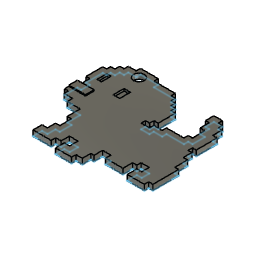
pixel_art_dog_keychain (Autodesk Fusion 360 design; units mm, degrees)
Autodesk Fusion 360 part; units mm, degrees
sketch "Dog_body" plane through (0, 0, 0) normal (0, 0, 1) x (1, 0, 0)
  line L0 (-5.9546, 3.7769) -> (-5.6, 3.7769)
  line L1 (-5.6, 3.7769) -> (-5.6, 4.1551)
  line L2 (-5.6, 4.1551) -> (-5.2, 4.1551)
  line L3 (-5.2, 4.1551) -> (-5.2, 4.6)
  line L4 (-5.2, 4.6) -> (-4.8, 4.6)
  line L5 (-4.8, 4.6) -> (-4.8, 5)
  line L6 (-4.8, 5) -> (-4.0585, 5)
  line L7 (-4.0585, 5) -> (-4.0585, 5.4)
  line L8 (-4.0585, 5.4) -> (-2.4, 5.4)
  line L9 (-2.4, 5.4) -> (-2.4, 5)
  line L10 (-2.4, 5) -> (-0.4, 5)
  line L11 (-0.4, 5) -> (-0.4, 4.6)
  line L12 (-5.9546, 3.7769) -> (-5.9546, 2.2)
  line L13 (-5.9546, 2.2) -> (-5.6, 2.2)
  line L14 (-5.6, 2.2) -> (-5.6, 1.4)
  line L15 (-5.6, 1.4) -> (-5.9546, 1.4)
  line L16 (-5.9546, 1.4) -> (-5.9546, 0.2)
  line L17 (-5.9546, 0.2) -> (-5.6, 0.2)
  line L18 (-5.6, 0.2) -> (-5.6, -0.2)
  line L19 (-5.6, -0.2) -> (-4.8, -0.2)
  line L20 (-4.8, -0.2) -> (-4.8, -0.7)
  line L21 (-4.8, -0.7) -> (-3.6, -0.7)
  line L22 (-3.6, -0.7) -> (-3.6, -1.9)
  line L23 (-3.6, -1.9) -> (-3.2, -1.9)
  line L24 (-3.2, -1.9) -> (-3.2, -3)
  line L25 (-3.2, -3) -> (-3.6, -3)
  line L26 (-3.6, -3) -> (-3.6, -3.7529)
  line L27 (-3.6, -3.7529) -> (-4.1, -3.7529)
  line L28 (-4.1, -3.7529) -> (-4.1, -4.6)
  line L29 (-4.1, -4.6) -> (-2.4, -4.6)
  line L30 (-2.4, -4.6) -> (-2.4, -4.1765)
  line L31 (-2.4, -4.1765) -> (-1.9, -4.1765)
  line L32 (-1.9, -4.1765) -> (-1.9, -3.4)
  line L33 (-1.9, -3.4) -> (-1.1, -3.4)
  line L34 (-1.1, -3.4) -> (-1.1, -4.1765)
  line L35 (-1.1, -4.1765) -> (-1.6, -4.1765)
  line L36 (-1.6, -4.1765) -> (-1.6, -5)
  line L37 (-1.6, -5) -> (-0.1, -5)
  line L38 (-0.1, -5) -> (-0.1, -4.5882)
  line L39 (-0.1, -4.5882) -> (0.5, -4.5882)
  line L40 (0.5, -4.5882) -> (0.5, -3.8)
  line L41 (5.1495, 3.3539) -> (5.1495, 1.4)
  line L42 (5.1495, 1.4) -> (4.8, 1.4)
  line L43 (4.8, 1.4) -> (4.8, 1)
  line L44 (4.8, 1) -> (5.1495, 1)
  line L45 (5.1495, 1) -> (5.1495, 0.2)
  line L46 (5.1495, 0.2) -> (5.5479, 0.2)
  line L47 (5.5479, 0.2) -> (5.5479, -1)
  line L48 (5.5479, -1) -> (5.9, -1)
  line L49 (5.9, -1) -> (5.9, -3.4)
  line L50 (-0.4, 4.6) -> (0, 4.6)
  line L51 (0, 4.6) -> (0, 4.2)
  line L52 (0, 4.2) -> (0.4, 4.2)
  line L53 (0.4, 4.2) -> (0.4, 3.8)
  line L54 (0.4, 3.8) -> (0.8, 3.8)
  line L55 (0.8, 3.8) -> (0.8, 3.4)
  line L56 (0.8, 3.4) -> (1.2, 3.4)
  line L57 (1.2, 3.4) -> (1.2, 1.8)
  line L58 (1.2, 1.8) -> (0.8, 1.8)
  line L59 (0.8, 1.8) -> (0.8, 1.4)
  line L60 (0.8, 1.4) -> (0.4, 1.4)
  line L61 (0.4, 1.4) -> (0.4, 1)
  line L62 (0.4, 1) -> (1.1786, 1)
  line L63 (1.1786, 1) -> (1.1786, 1.4)
  line L64 (1.1786, 1.4) -> (1.9689, 1.4)
  line L65 (1.9689, 1.4) -> (1.9689, 1.8)
  line L66 (1.9689, 1.8) -> (3.6, 1.8)
  line L67 (3.6, 1.8) -> (3.6, 2.2)
  line L68 (3.6, 2.2) -> (4, 2.2)
  line L69 (4, 2.2) -> (4, 3.3596)
  line L70 (4, 3.3596) -> (3.5503, 3.3596)
  line L71 (3.5503, 3.3596) -> (3.5503, 4.2)
  line L72 (3.5503, 4.2) -> (3.2, 4.2)
  line L73 (3.2, 4.2) -> (3.2, 5)
  line L74 (3.2, 5) -> (4, 5)
  line L75 (4, 5) -> (4, 4.6)
  line L76 (4, 4.6) -> (4.4, 4.6)
  line L77 (4.4, 4.6) -> (4.4, 4.2)
  line L78 (4.4, 4.2) -> (4.7373, 4.2)
  line L79 (4.7373, 4.2) -> (4.7373, 3.4)
  line L80 (4.7373, 3.4) -> (4.7373, 3.3539)
  line L81 (4.7373, 3.3539) -> (5.1495, 3.3539)
  line L82 (0.5, -3.8) -> (0.8, -3.8)
  line L83 (0.8, -3.8) -> (0.8, -3)
  line L84 (0.8, -3) -> (1.5654, -3)
  line L85 (1.5654, -3) -> (1.5654, -3.5)
  line L86 (1.5654, -3.5) -> (3.2, -3.5)
  line L87 (3.2, -3.5) -> (3.2, -2.6)
  line L88 (3.2, -2.6) -> (3.6, -2.6)
  line L89 (3.6, -2.6) -> (3.6, -2.2)
  line L90 (3.6, -2.2) -> (4.3564, -2.2)
  line L91 (4.3564, -2.2) -> (4.3564, -2.9)
  line L92 (4.3564, -2.9) -> (3.9, -2.9)
  line L93 (3.9, -2.9) -> (3.9, -3.8)
  line L94 (3.9, -3.8) -> (5.5, -3.8)
  line L95 (5.5, -3.4) -> (5.9, -3.4)
  line L96 (5.5, -3.4) -> (5.5, -3.8)
  constraint horizontal L0
  constraint perpendicular L0 L1
  constraint perpendicular L1 L2
  constraint perpendicular L2 L3
  constraint perpendicular L3 L4
  constraint perpendicular L4 L5
  constraint perpendicular L3 L6
  constraint perpendicular L6 L7
  constraint perpendicular L7 L8
  constraint perpendicular L8 L9
  constraint perpendicular L9 L10
  constraint perpendicular L10 L11
  constraint perpendicular L0 L12
  constraint perpendicular L12 L13
  constraint perpendicular L0 L14
  constraint perpendicular L14 L15
  constraint perpendicular L0 L16
  constraint perpendicular L14 L17
  constraint perpendicular L0 L18
  constraint perpendicular L18 L19
  constraint perpendicular L19 L20
  constraint perpendicular L20 L21
  constraint perpendicular L21 L22
  constraint perpendicular L22 L23
  constraint perpendicular L23 L24
  constraint perpendicular L24 L25
  constraint perpendicular L25 L26
  constraint perpendicular L24 L27
  constraint perpendicular L27 L28
  constraint perpendicular L28 L29
  constraint perpendicular L29 L30
  constraint perpendicular L30 L31
  constraint perpendicular L31 L32
  constraint perpendicular L32 L33
  constraint perpendicular L31 L34
  constraint perpendicular L34 L35
  constraint perpendicular L35 L36
  constraint perpendicular L36 L37
  constraint perpendicular L37 L38
  constraint perpendicular L38 L39
  constraint perpendicular L39 L40
  constraint vertical L41
  constraint perpendicular L41 L42
  constraint perpendicular L42 L43
  constraint perpendicular L43 L44
  constraint perpendicular L44 L45
  constraint perpendicular L45 L46
  constraint perpendicular L46 L47
  constraint perpendicular L47 L48
  constraint perpendicular L46 L49
  constraint perpendicular L11 L50
  constraint perpendicular L50 L51
  constraint perpendicular L51 L52
  constraint perpendicular L52 L53
  constraint perpendicular L53 L54
  constraint perpendicular L52 L55
  constraint perpendicular L55 L56
  constraint perpendicular L56 L57
  constraint perpendicular L57 L58
  constraint perpendicular L58 L59
  constraint perpendicular L59 L60
  constraint perpendicular L60 L61
  constraint perpendicular L59 L62
  constraint perpendicular L62 L63
  constraint perpendicular L63 L64
  constraint perpendicular L62 L65
  constraint perpendicular L65 L66
  constraint perpendicular L66 L67
  constraint perpendicular L67 L68
  constraint perpendicular L68 L69
  constraint perpendicular L67 L70
  constraint perpendicular L70 L71
  constraint perpendicular L71 L72
  constraint perpendicular L72 L73
  constraint perpendicular L73 L74
  constraint perpendicular L72 L75
  constraint perpendicular L75 L76
  constraint perpendicular L76 L77
  constraint perpendicular L77 L78
  constraint perpendicular L76 L79
  constraint perpendicular L76 L80
  constraint perpendicular L41 L81
  constraint perpendicular L40 L82
  constraint perpendicular L82 L83
  constraint perpendicular L83 L84
  constraint perpendicular L84 L85
  constraint perpendicular L85 L86
  constraint perpendicular L86 L87
  constraint perpendicular L87 L88
  constraint perpendicular L86 L89
  constraint perpendicular L89 L90
  constraint perpendicular L86 L91
  constraint perpendicular L91 L92
  constraint perpendicular L92 L93
  constraint perpendicular L91 L94
  constraint perpendicular L49 L95
  constraint perpendicular L94 L96
extrude "Extrude1" add sketch "Dog_body" along normal blind 0.5
sketch "Dog_eyes" plane through (0, 0, 0.5) normal (0, 0, 1) x (-1, 0, 0)
  line L0 (5.9546, -3.7769) -> (5.9546, -2.2)
  line L1 (5.9546, -2.2) -> (5.6, -2.2)
  line L2 (5.6, -2.2) -> (5.6, -1.4)
  line L3 (5.6, -1.4) -> (5.9546, -1.4)
  line L4 (5.9546, -1.4) -> (5.9546, -0.2)
  line L5 (5.9546, -0.2) -> (5.6, -0.2)
  line L6 (5.6, -0.2) -> (5.6, 0.2)
  line L7 (5.6, 0.2) -> (4.8, 0.2)
  line L8 (4.8, 0.2) -> (4.8, 0.7)
  line L9 (4.8, 0.7) -> (3.6, 0.7)
  line L10 (3.6, 0.7) -> (3.6, 1.9)
  line L11 (3.6, 1.9) -> (3.2, 1.9)
  line L12 (3.2, 1.9) -> (3.2, 3)
  line L13 (3.2, 3) -> (3.6, 3)
  line L14 (3.6, 3) -> (3.6, 3.7529)
  line L15 (3.6, 3.7529) -> (4.1, 3.7529)
  line L16 (4.1, 3.7529) -> (4.1, 4.6)
  line L17 (4.1, 4.6) -> (2.4, 4.6)
  line L18 (2.4, 4.6) -> (2.4, 4.1765)
  line L19 (2.4, 4.1765) -> (1.9, 4.1765)
  line L20 (1.9, 4.1765) -> (1.9, 3.4)
  line L21 (1.9, 3.4) -> (1.1, 3.4)
  line L22 (1.1, 3.4) -> (1.1, 4.1765)
  line L23 (1.1, 4.1765) -> (1.6, 4.1765)
  line L24 (1.6, 4.1765) -> (1.6, 5)
  line L25 (1.6, 5) -> (0.1, 5)
  line L26 (0.1, 5) -> (0.1, 4.5882)
  line L27 (0.1, 4.5882) -> (-0.5, 4.5882)
  line L28 (-0.5, 4.5882) -> (-0.5, 3.8)
  line L29 (-0.5, 3.8) -> (-0.8, 3.8)
  line L30 (-0.8, 3.8) -> (-0.8, 3)
  line L31 (-0.8, 3) -> (-1.5654, 3)
  line L32 (-1.5654, 3) -> (-1.5654, 3.5)
  line L33 (-1.5654, 3.5) -> (-3.2, 3.5)
  line L34 (-3.2, 3.5) -> (-3.2, 2.6)
  line L35 (-3.2, 2.6) -> (-3.6, 2.6)
  line L36 (-3.6, 2.6) -> (-3.6, 2.2)
  line L37 (-3.6, 2.2) -> (-4.3564, 2.2)
  line L38 (-4.3564, 2.2) -> (-4.3564, 2.9)
  line L39 (-4.3564, 2.9) -> (-3.9, 2.9)
  line L40 (-3.9, 2.9) -> (-3.9, 3.8)
  line L41 (-3.9, 3.8) -> (-5.5, 3.8)
  line L42 (-5.5, 3.8) -> (-5.5, 3.4)
  line L43 (-5.5, 3.4) -> (-5.9, 3.4)
  line L44 (-5.9, 3.4) -> (-5.9, 1)
  line L45 (-5.9, 1) -> (-5.5479, 1)
  line L46 (-5.5479, 1) -> (-5.5479, -0.2)
  line L47 (-5.5479, -0.2) -> (-5.1495, -0.2)
  line L48 (-5.1495, -0.2) -> (-5.1495, -1)
  line L49 (-5.1495, -1) -> (-4.8, -1)
  line L50 (-4.8, -1) -> (-4.8, -1.4)
  line L51 (-4.8, -1.4) -> (-5.1495, -1.4)
  line L52 (-5.1495, -1.4) -> (-5.1495, -3.3539)
  line L53 (-5.1495, -3.3539) -> (-4.7373, -3.3539)
  line L54 (-4.7373, -3.3539) -> (-4.7373, -4.2)
  line L55 (-4.7373, -4.2) -> (-4.4, -4.2)
  line L56 (-4.4, -4.2) -> (-4.4, -4.6)
  line L57 (-4.4, -4.6) -> (-4, -4.6)
  line L58 (-4, -4.6) -> (-4, -5)
  line L59 (-4, -5) -> (-3.2, -5)
  line L60 (-3.2, -5) -> (-3.2, -4.2)
  line L61 (-3.2, -4.2) -> (-3.5503, -4.2)
  line L62 (-3.5503, -4.2) -> (-3.5503, -3.3596)
  line L63 (-3.5503, -3.3596) -> (-4, -3.3596)
  line L64 (-4, -3.3596) -> (-4, -2.2)
  line L65 (-4, -2.2) -> (-3.6, -2.2)
  line L66 (-3.6, -2.2) -> (-3.6, -1.8)
  line L67 (-3.6, -1.8) -> (-1.9689, -1.8)
  line L68 (-1.9689, -1.8) -> (-1.9689, -1.4)
  line L69 (-1.9689, -1.4) -> (-1.1786, -1.4)
  line L70 (-1.1786, -1.4) -> (-1.1786, -1)
  line L71 (-1.1786, -1) -> (-0.4, -1)
  line L72 (-0.4, -1) -> (-0.4, -1.4)
  line L73 (-0.4, -1.4) -> (-0.8, -1.4)
  line L74 (-0.8, -1.4) -> (-0.8, -1.8)
  line L75 (-0.8, -1.8) -> (-1.2, -1.8)
  line L76 (-1.2, -1.8) -> (-1.2, -3.4)
  line L77 (-1.2, -3.4) -> (-0.8, -3.4)
  line L78 (-0.8, -3.4) -> (-0.8, -3.8)
  line L79 (-0.8, -3.8) -> (-0.4, -3.8)
  line L80 (-0.4, -3.8) -> (-0.4, -4.2)
  line L81 (-0.4, -4.2) -> (0, -4.2)
  line L82 (0, -4.2) -> (0, -4.6)
  line L83 (0, -4.6) -> (0.4, -4.6)
  line L84 (0.4, -4.6) -> (0.4, -5)
  line L85 (0.4, -5) -> (2.4, -5)
  line L86 (2.4, -5) -> (2.4, -5.4)
  line L87 (2.4, -5.4) -> (4.0585, -5.4)
  line L88 (4.0585, -5.4) -> (4.0585, -5)
  line L89 (4.0585, -5) -> (4.8, -5)
  line L90 (4.8, -5) -> (4.8, -4.6)
  line L91 (4.8, -4.6) -> (5.2, -4.6)
  line L92 (5.2, -4.6) -> (5.2, -4.1551)
  line L93 (5.2, -4.1551) -> (5.6, -4.1551)
  line L94 (5.6, -4.1551) -> (5.6, -3.7769)
  line L95 (5.6, -3.7769) -> (5.9546, -3.7769)
  line L96 (3.2, -3) -> (3.2, -2)
  line L97 (3.2, -2) -> (2.6, -2)
  line L98 (2.6, -2) -> (2.6, -3)
  line L99 (2.6, -3) -> (3.2, -3)
  line L100 (5.2, -3.3) -> (5.2, -2.5)
  line L101 (5.2, -2.5) -> (4.8, -2.5)
  line L102 (4.8, -2.5) -> (4.8, -3.4)
  line L103 (4.8, -3.4) -> (5.2, -3.4)
  line L104 (5.2, -3.4) -> (5.2, -3.3)
  constraint vertical L96
  constraint perpendicular L96 L97
  constraint perpendicular L97 L98
  constraint perpendicular L96 L99
  constraint perpendicular L99 L100
  constraint perpendicular L96 L101
  constraint perpendicular L101 L102
  constraint perpendicular L102 L103
  constraint perpendicular L103 L104
extrude "Extrude2" cut sketch "Dog_eyes" against normal blind 0.2 contours L96 L97 L98 L99 | L100 L101 L102 L103 L104
sketch "Sketch3" plane through (0, 0, 0.5) normal (0, 0, 1) x (-1, 0, 0)
  line L0 (4.8, -2.5) -> (5.2, -2.5)
  line L1 (5.2, -2.5) -> (5.2, -3.4)
  line L2 (5.2, -3.4) -> (4.8, -3.4)
  line L3 (4.8, -3.4) -> (4.8, -2.5)
  line L4 (3.2, -2) -> (3.2, -3)
  line L5 (3.2, -3) -> (2.6, -3)
  line L6 (2.6, -3) -> (2.6, -2)
  line L7 (2.6, -2) -> (3.2, -2)
  line L8 (5.9546, -3.7769) -> (5.9546, -2.2)
  line L9 (5.9546, -2.2) -> (5.6, -2.2)
  line L10 (5.6, -2.2) -> (5.6, -1.4)
  line L11 (5.6, -1.4) -> (5.9546, -1.4)
  line L12 (5.9546, -1.4) -> (5.9546, -0.2)
  line L13 (5.9546, -0.2) -> (5.6, -0.2)
  line L14 (5.6, -0.2) -> (5.6, 0.2)
  line L15 (5.6, 0.2) -> (4.8, 0.2)
  line L16 (4.8, 0.2) -> (4.8, 0.7)
  line L17 (4.8, 0.7) -> (3.6, 0.7)
  line L18 (3.6, 0.7) -> (3.6, 1.9)
  line L19 (3.6, 1.9) -> (3.2, 1.9)
  line L20 (3.2, 1.9) -> (3.2, 3)
  line L21 (3.2, 3) -> (3.6, 3)
  line L22 (3.6, 3) -> (3.6, 3.7529)
  line L23 (3.6, 3.7529) -> (4.1, 3.7529)
  line L24 (4.1, 3.7529) -> (4.1, 4.6)
  line L25 (4.1, 4.6) -> (2.4, 4.6)
  line L26 (2.4, 4.6) -> (2.4, 4.1765)
  line L27 (2.4, 4.1765) -> (1.9, 4.1765)
  line L28 (1.9, 4.1765) -> (1.9, 3.4)
  line L29 (1.9, 3.4) -> (1.1, 3.4)
  line L30 (1.1, 3.4) -> (1.1, 4.1765)
  line L31 (1.1, 4.1765) -> (1.6, 4.1765)
  line L32 (1.6, 4.1765) -> (1.6, 5)
  line L33 (1.6, 5) -> (0.1, 5)
  line L34 (0.1, 5) -> (0.1, 4.5882)
  line L35 (0.1, 4.5882) -> (-0.5, 4.5882)
  line L36 (-0.5, 4.5882) -> (-0.5, 3.8)
  line L37 (-0.5, 3.8) -> (-0.8, 3.8)
  line L38 (-0.8, 3.8) -> (-0.8, 3)
  line L39 (-0.8, 3) -> (-1.5654, 3)
  line L40 (-1.5654, 3) -> (-1.5654, 3.5)
  line L41 (-1.5654, 3.5) -> (-3.2, 3.5)
  line L42 (-3.2, 3.5) -> (-3.2, 2.6)
  line L43 (-3.2, 2.6) -> (-3.6, 2.6)
  line L44 (-3.6, 2.6) -> (-3.6, 2.2)
  line L45 (-3.6, 2.2) -> (-4.3564, 2.2)
  line L46 (-4.3564, 2.2) -> (-4.3564, 2.9)
  line L47 (-4.3564, 2.9) -> (-3.9, 2.9)
  line L48 (-3.9, 2.9) -> (-3.9, 3.8)
  line L49 (-3.9, 3.8) -> (-5.5, 3.8)
  line L50 (-5.5, 3.8) -> (-5.5, 3.4)
  line L51 (-5.5, 3.4) -> (-5.9, 3.4)
  line L52 (-5.9, 3.4) -> (-5.9, 1)
  line L53 (-5.9, 1) -> (-5.5479, 1)
  line L54 (-5.5479, 1) -> (-5.5479, -0.2)
  line L55 (-5.5479, -0.2) -> (-5.1495, -0.2)
  line L56 (-5.1495, -0.2) -> (-5.1495, -1)
  line L57 (-5.1495, -1) -> (-4.8, -1)
  line L58 (-4.8, -1) -> (-4.8, -1.4)
  line L59 (-4.8, -1.4) -> (-5.1495, -1.4)
  line L60 (-5.1495, -1.4) -> (-5.1495, -3.3539)
  line L61 (-5.1495, -3.3539) -> (-4.7373, -3.3539)
  line L62 (-4.7373, -3.3539) -> (-4.7373, -4.2)
  line L63 (-4.7373, -4.2) -> (-4.4, -4.2)
  line L64 (-4.4, -4.2) -> (-4.4, -4.6)
  line L65 (-4.4, -4.6) -> (-4, -4.6)
  line L66 (-4, -4.6) -> (-4, -5)
  line L67 (-4, -5) -> (-3.2, -5)
  line L68 (-3.2, -5) -> (-3.2, -4.2)
  line L69 (-3.2, -4.2) -> (-3.5503, -4.2)
  line L70 (-3.5503, -4.2) -> (-3.5503, -3.3596)
  line L71 (-3.5503, -3.3596) -> (-4, -3.3596)
  line L72 (-4, -3.3596) -> (-4, -2.2)
  line L73 (-4, -2.2) -> (-3.6, -2.2)
  line L74 (-3.6, -2.2) -> (-3.6, -1.8)
  line L75 (-3.6, -1.8) -> (-1.9689, -1.8)
  line L76 (-1.9689, -1.8) -> (-1.9689, -1.4)
  line L77 (-1.9689, -1.4) -> (-1.1786, -1.4)
  line L78 (-1.1786, -1.4) -> (-1.1786, -1)
  line L79 (-1.1786, -1) -> (-0.4, -1)
  line L80 (-0.4, -1) -> (-0.4, -1.4)
  line L81 (-0.4, -1.4) -> (-0.8, -1.4)
  line L82 (-0.8, -1.4) -> (-0.8, -1.8)
  line L83 (-0.8, -1.8) -> (-1.2, -1.8)
  line L84 (-1.2, -1.8) -> (-1.2, -3.4)
  line L85 (-1.2, -3.4) -> (-0.8, -3.4)
  line L86 (-0.8, -3.4) -> (-0.8, -3.8)
  line L87 (-0.8, -3.8) -> (-0.4, -3.8)
  line L88 (-0.4, -3.8) -> (-0.4, -4.2)
  line L89 (-0.4, -4.2) -> (0, -4.2)
  line L90 (0, -4.2) -> (0, -4.6)
  line L91 (0, -4.6) -> (0.4, -4.6)
  line L92 (0.4, -4.6) -> (0.4, -5)
  line L93 (0.4, -5) -> (2.4, -5)
  line L94 (2.4, -5) -> (2.4, -5.4)
  line L95 (2.4, -5.4) -> (4.0585, -5.4)
  line L96 (4.0585, -5.4) -> (4.0585, -5)
  line L97 (4.0585, -5) -> (4.8, -5)
  line L98 (4.8, -5) -> (4.8, -4.6)
  line L99 (4.8, -4.6) -> (5.2, -4.6)
  line L100 (5.2, -4.6) -> (5.2, -4.1551)
  line L101 (5.2, -4.1551) -> (5.6, -4.1551)
  line L102 (5.6, -4.1551) -> (5.6, -3.7769)
  line L103 (5.6, -3.7769) -> (5.9546, -3.7769)
  line L104 (5.6, -1.4) -> (4.4, -1.4)
  line L105 (4.4, -1.4) -> (4.4, -0.6)
  line L106 (4.4, -0.6) -> (5.9546, -0.6)
  line L107 (5.9546, -1.4) -> (5.5, -1.4)
  line L108 (5.6, -1.4) -> (5.9546, -1.4)
  line L109 (5.6, -1.4) -> (4.4, -1.4)
  line L110 (5.6, -1.4) -> (5.9546, -1.4)
  line L111 (5.9546, -0.6568) -> (5.9546, -0.6)
  line L112 (5.9546, -0.6) -> (5.9546, -1.4)
  constraint coincident L10.end L11.start
  constraint perpendicular L12 L104
  constraint perpendicular L104 L105
  constraint coincident L12 L106.end
  constraint perpendicular L12 L106
  constraint coincident L11.end L12.start
  constraint coincident L104 L107.end
  constraint perpendicular L10 L107
  constraint coincident L12 L111.start
extrude "Extrude3" add sketch "Sketch3" along normal blind 0.2 contours L11 L12 L104 L105 L106 L107 L108 L109 L110 L111 L112
extrude "Extrude4" cut 1 faces at (-4.9182, 0.8667, 0.7) along direction (0, 0, -1) blind 0.1
hole "Hole1" at (-3.4028, 4.5934, 0.5) direction (0, 0, -1) diameter 1 depth 2.5 tip angle 118
named bodies: "Dog_Body"
